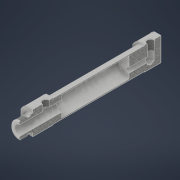
# Autodesk Inventor part: 8112003 DSNU-S-12-30-P-MQ---(C)
Saved by Autodesk Inventor 2022 (Build 260153000, 153)
## iProperties
Created: 2023-03-28
Part Number: 8112003 DSNU-S-12-30-P-MQ---(C)
Material: Generic
Catalog Web Link: www.cadenas.de
Description: DSNU-S---(C)-ISO cylinder
Vendor: FESTO
Document SubType Name: Modeling
Designer: psAdmin
Manufacturer: FESTO
Mass: 6.57651 g
Surface Area: 63.4029 cm^2
Volume: 6.57651 cm^3
Density: 1 g/cm^3
Appearance: PSOLRGB-175-175-175
Category: PARTsolutions
Company: FESTO
PSOL_IDENT_0: {$CADENAS_DATA/23d-libs/festo/parts/d/dsnu/parts/dsnu_s_cylinder.prj},218 {VTYP=3D},{NB=8112003 DSNU
PSOL_IDENT_1: -S-12-30-P-MQ---(C)},{LINA=8112003 DSNU-S-12-30-P-MQ},{NN=DSNU-S---(C)},{DATE=13.03.2023 13:59:39},{
PSOL_IDENT_2: GEOMDATE=27.10.2022 12:31:00},{VERSION=},{LINEID=30},{WBVAR=HUB,DA,PE,ZYL},{WBNUMERIC=HUB}  {NB=8112
PSOL_IDENT_3: 003 DSNU-S-12-30-P-MQ---(C)},{LINA=8112003 DSNU-S-12-30-P-MQ},{KT=DUMMY},{TNR=8112003},{TYP=DSNU-S-1
PSOL_IDENT_4: 2},{KDM=12},{HUB=30},{DA=P},{DA1='P'},{PE=-},{PE1=},{BWE=-},{BWE1=},{ZYL=MQ},{AM=16},{B=10},{BE=M10x
PSOL_IDENT_5: 1},{BEM=10},{BEP=1.000},{BF=8.1},{D1=14},{D4=13.3},{EE=M5},{EEM=5.000},{G=9.65},{G1=11.95},{KK=M6},{
PSOL_IDENT_6: KKM=6},{KV=14},{KW=4},{L2=75.85},{MM=6},{PL=6.0},{PL1=8.0},{VD=1.5},{WF=13.0},{ZJ=89.3},{BEM1=8.400}
PSOL_IDENT_7: ,{BER=0.600},{BEL=3.000},{KKL=3.600},{EEL=4.000},{D5=16.0},{ZYLT=-MQ}
NB: 8112003 DSNU-S-12-30-P-MQ---(C)
NN: DSNU-S---(C)
NT: ISO cylinder
NBSYN: $TNR. $TYP.-$HUB.-$DA.$PE1.$BWE1.$ZYLT.---(C)
LINA: 8112003 DSNU-S-12-30-P-MQ
CATALOG: Festo
TNR: 8112003
TYP: DSNU-S-12
KDM: 12
HUB: 30
DA: P
DA1: 'P'
PE: -
BWE: -
ZYL: MQ
AM: 16
B: 10
BE: M10x1
BEM: 10
BEP: 1
BF: 8.1
D1: 14
D4: 13.3
EE: M5
EEM: 5
KK: M6
KKM: 6
KV: 14
KW: 4
MM: 6
PL: 6
PL1: 8
VD: 1.5
WF: 13
BEM1: 8.4
BER: 0.6
BEL: 3
KKL: 3.6
EEL: 4
D5: 16
SUPPLIER: FESTO
ARTICLENO: 8112003 DSNU-S-12-30-P-MQ---(C)
BOMINFO: 8112003 DSNU-S-12-30-P-MQ
CREATOR: CADENAS GmbH
Title: 8112003 DSNU-S-12-30-P-MQ
Author: Cadenas PARTsolutions
Comments: ISO cylinder
Autodesk Inventor part; units mm, degrees
sketch "Sketch_12" plane through (0, 0, 0) normal (1, 0, 0) x (0, 1, 0)
  line L0 (0, -75.85) -> (0, 0)
  line L1 (0, 0) -> (8, 0)
  line L2 (8, 0) -> (8, -11.95)
  line L3 (8, -11.95) -> (6.65, -11.95)
  line L4 (6.65, -11.95) -> (6.65, -66.2)
  line L5 (6.65, -66.2) -> (8, -66.2)
  line L6 (8, -66.2) -> (8, -75.85)
  line L7 (8, -75.85) -> (0, -75.85)
  line L8 (0, -75.85) -> (0, 0)
  constraints: 18 end point
revolve "Revolution1" add sketch "Sketch_12" angle 360 about axis through (0, 0, -75.85) along (0, 0, -1)
sketch "Sketch_3" plane through (0, 0, 0) normal (1, 0, 0) x (0, 1, 0)
  line L0 (0, 0) -> (0, 8.1)
  line L1 (0, 8.1) -> (4.3865, 8.1)
  line L2 (4.3865, 8.1) -> (5, 7.4865)
  line L3 (5, 7.4865) -> (5, 3.6135)
  line L4 (5, 3.6135) -> (4.3757, 2.9892)
  arc A0 (4.3757, 2.9892) -> (4.2, 2.565) centre (4.8, 2.565) ccw
  line L5 (4.2, 2.565) -> (4.2, 2.2)
  arc A1 (4.2, 2.2) -> (4.8, 1.6) centre (4.8, 2.2) ccw
  line L6 (4.8, 1.6) -> (5, 1.6)
  line L7 (5, 1.6) -> (5, 0)
  line L8 (5, 0) -> (0, 0)
  line L9 (0, 0) -> (0, 8.1)
  constraints: 20 end point, 4 point on circle, 2 centre point
revolve "Revolution2" add sketch "Sketch_3" angle 360 about axis through (0, 0, 0) along (0, 0, -1)
thread "Thread1" size "M10x1" class "6g" standard "ISO Metric profile" full length
sketch "Sketch_7" plane through (0, 0, 0) normal (0, 0, 1) x (1, 0, 0)
  line L0 (-14, 14) -> (-14, -14)
  line L1 (-14, -14) -> (14, -14)
  line L2 (14, -14) -> (14, 14)
  line L3 (14, 14) -> (-14, 14)
  line L4 (-7, 7) -> (-7, -7)
  line L5 (-7, -7) -> (7, -7)
  line L6 (7, -7) -> (7, 7)
  line L7 (7, 7) -> (-7, 7)
  constraints: 16 end point
extrude "Extrusion1" cut sketch "Sketch_7" against normal blind 75.85
sketch "Sketch4" plane through (-3.873, 7, -11.95) normal (0, 1, 0) x (1, 0, 0)
  point P0 (3.873, -3.95)
hole "Hole1" at (0, 7, -8) direction (0, -1, 0) diameter 4.134 depth 7 countersink diameter 5 countersink angle 90 thread size "M5x0.8" class "6H" standard "ISO Metric profile"
sketch "Sketch5" plane through (-3.873, 7, -66.2) normal (0, 1, 0) x (1, 0, 0)
  point P0 (3.873, 3.65)
hole "Hole2" at (0, 7, -69.85) direction (0, -1, 0) diameter 4.134 depth 11 tip angle 120 countersink diameter 5 countersink angle 90 thread size "M5x0.8" class "6H" standard "ISO Metric profile"
sketch "Sketch_10" plane through (0, 0, 0) normal (1, 0, 0) x (0, 1, 0)
  line L0 (0, -57) -> (0, 8.1)
  line L1 (0, 8.1) -> (3.4, 8.1)
  line L2 (3.4, 8.1) -> (3, 7.7)
  line L3 (3, 7.7) -> (3, -17)
  line L4 (3, -17) -> (6, -17)
  line L5 (6, -17) -> (6, -57)
  line L6 (6, -57) -> (0, -57)
  line L7 (0, -57) -> (0, 8.1)
  constraints: 16 end point
revolve "Revolution3" cut sketch "Sketch_10" angle 360 about axis through (0, 0, -57) along (0, 0, -1)
ref_plane "ANBAU_XY" through (0, 0, 0) normal (0, 0, 1) x (1, 0, 0)
ref_plane "ANBAU_YZ" through (0, 0, 0) normal (1, 0, 0) x (0, 1, 0)
ref_plane "ANBAU_ZX" through (0, 0, 0) normal (0, 1, 0) x (0, 0, 1)
ref_plane "FDT_FRONT_XY" through (0, 0, 0) normal (0, 0, -1) x (-1, 0, 0)
ref_plane "FDT_FRONT_YZ" through (0, 0, 0) normal (-1, 0, 0) x (0, 1, 0)
ref_plane "FDT_FRONT_ZX" through (0, 0, 0) normal (0, 1, 0) x (0, 0, -1)
ref_plane "FDT_QSFRONT_XY" through (0, 7, -8) normal (0, 1, 0) x (1, 0, 0)
ref_plane "FDT_QSFRONT_YZ" through (0, 7, -8) normal (1, 0, 0) x (0, 0, -1)
ref_plane "FDT_QSFRONT_ZX" through (0, 7, -8) normal (0, 0, -1) x (0, 1, 0)
ref_plane "FDT_QSREAR_XY" through (0, 7, -69.85) normal (0, 1, 0) x (1, 0, 0)
ref_plane "FDT_QSREAR_YZ" through (0, 7, -69.85) normal (1, 0, 0) x (0, 0, -1)
ref_plane "FDT_QSREAR_ZX" through (0, 7, -69.85) normal (0, 0, -1) x (0, 1, 0)
ref_plane "FDT_REAR_XY" through (0, 0, -75.85) normal (0, 0, 1) x (-1, 0, 0)
ref_plane "FDT_REAR_YZ" through (0, 0, -75.85) normal (-1, 0, 0) x (0, -1, 0)
ref_plane "FDT_REAR_ZX" through (0, 0, -75.85) normal (0, -1, 0) x (0, 0, 1)
ref_plane "FDT_SMBR1_XY" through (0, 0, -21.45) normal (0, 0, 1) x (1, 0, 0)
ref_plane "FDT_SMBR1_YZ" through (0, 0, -21.45) normal (1, 0, 0) x (0, 1, 0)
ref_plane "FDT_SMBR1_ZX" through (0, 0, -21.45) normal (0, 1, 0) x (0, 0, 1)
ref_plane "FDT_SMBR2_XY" through (0, 0, -56.7) normal (0, 0, 1) x (1, 0, 0)
ref_plane "FDT_SMBR2_YZ" through (0, 0, -56.7) normal (1, 0, 0) x (0, 1, 0)
ref_plane "FDT_SMBR2_ZX" through (0, 0, -56.7) normal (0, 1, 0) x (0, 0, 1)
ref_plane "to_nut_XY" through (0, 0, 3.6) normal (0, 0, 1) x (1, 0, 0)
ref_plane "to_nut_YZ" through (0, 0, 3.6) normal (1, 0, 0) x (0, 1, 0)
ref_plane "to_nut_ZX" through (0, 0, 3.6) normal (0, 1, 0) x (0, 0, 1)
ref_plane "to_piston_XY" through (0, 0, -57) normal (0, 0, 1) x (1, 0, 0)
ref_plane "to_piston_YZ" through (0, 0, -57) normal (1, 0, 0) x (0, 1, 0)
ref_plane "to_piston_ZX" through (0, 0, -57) normal (0, 1, 0) x (0, 0, 1)
sketch "Szkic7" plane through (0, 0, -17) normal (0, 0, -1) x (-1, 0, 0)
  circle A0 centre (0, 2.745) radius 0.5831
  point P0 (0, 0)
  constraints: 1 centre point
extrude "Wyciągnięcie proste2" cut sketch "Szkic7" against normal blind 9.5
sketch "Szkic8" plane through (0, 0, -57) normal (0, 0, 1) x (1, 0, 0)
  circle A0 centre (0, -1.5) radius 1.5
  point P0 (0, 0)
  constraints: 1 vertical alignment, 2 other
extrude "Wyciągnięcie proste3" cut sketch "Szkic8" against normal blind 12.5
body "Solid1"
